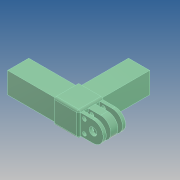
# Autodesk Inventor part: KB33-046-001-001 - Уголок
Saved by Autodesk Inventor 2020 (Build 240168000, 168)
## iProperties
Created: 2021-06-20
Part Number: KB33-046-001-001 - Уголок
Material: Пластик АБС
Document SubType Name: Modeling
Designer: Петров Иван
Mass: 150.443 g
Surface Area: 266.997 cm^2
Volume: 141.927 cm^3
Density: 1.06 g/cm^3
Appearance: Гладкий — темный цвет морской волны
Author: Петров Иван
Autodesk Inventor part; units mm, degrees
ref_plane "YZ Plane" through (0, 0, 0) normal (1, 0, 0) x (0, 1, 0)
ref_plane "XZ Plane" through (0, 0, 0) normal (0, 1, 0) x (-1, 0, 0)
ref_plane "XY Plane" through (0, 0, 0) normal (0, 0, 1) x (1, 0, 0)
sketch "Эскиз1" plane through (0, 0, 0) normal (0, 1, 0) x (-1, 0, 0)
  line L0 (-16, 16) -> (16, 16)
  line L1 (16, 16) -> (16, -16)
  line L2 (16, -16) -> (-16, -16)
  line L3 (-16, -16) -> (-16, 16)
  line L4 (-16, 16) -> (16, -16) construction
  line L5 (16, 16) -> (-16, -16) construction
  point P0 (0, 0)
  dimension "d0" = 32
  dimension "d1" = 32
  constraints: 12 end point, 2 midpoint, 2 parallel, 1 horizontal, 1 perpendicular
  measures "d0" distance of L1.end L2.end
  measures "d1" distance of L0.end L1.end
extrude "Выдавливание1" add sketch "Эскиз1" along normal blind 32
sketch "Эскиз2" plane through (16, 0, -16) normal (0, 0, -1) x (-1, 0, 0)
  line L0 (16, 0) -> (16, 16) construction
  line L1 (2, 2) -> (30, 2)
  line L2 (30, 2) -> (30, 30)
  line L3 (30, 30) -> (2, 30)
  line L4 (2, 30) -> (2, 2)
  line L5 (2, 2) -> (30, 30) construction
  line L6 (30, 2) -> (2, 30) construction
  dimension "d5" = 16
  dimension "d6" = 28
  dimension "d7" = 28
  constraints: 14 end point, 2 midpoint, 2 parallel, 1 horizontal, 1 perpendicular, 1 vertical
  measures "d5" distance of L0.start L0.end
  measures "d6" distance of L3.end L2.end
  measures "d7" distance of L2.end L1.end
extrude "Выдавливание2" add sketch "Эскиз2" along normal blind 64
pattern_circular "Круговой массив1" count 2 over 90 about axis through (0, -10, 0) along (0, 1, 0) of "Выдавливание2"
fillet "Сопряжение1" radius 2.5 5 edges at (16, 32, 0) (0, 32, 16) (0, 0, 16) (16, 0, 0) (16, 16, 16)
sketch "Эскиз5" plane through (16, 2.5, 13.5) normal (1, 0, 0) x (0, 0, -1)
  line L0 (0, 27) -> (29.5, 27) projected
  line L1 (0, 0) -> (0, 27) projected
  line L2 (29.5, 0) -> (0, 0) projected
  line L3 (29.5, 0) -> (29.5, 27) projected
  line L4 (0, 27) -> (29.5, 27) projected
  line L5 (29.5, 0) -> (0, 0) projected
  line L6 (0, 27) -> (4, 27)
  line L7 (4, 27) -> (4, 0)
  line L8 (4, 0) -> (0, 0)
  line L9 (0, 0) -> (0, 27)
  line L10 (29.5, 27) -> (25.5, 27)
  line L11 (25.5, 27) -> (25.5, 0)
  line L12 (25.5, 0) -> (29.5, 0)
  line L13 (29.5, 0) -> (29.5, 27)
  line L14 (10, 27) -> (19.5, 27)
  line L15 (19.5, 27) -> (19.5, 0)
  line L16 (19.5, 0) -> (10, 0)
  line L17 (10, 0) -> (10, 27)
  point P0 (13.5, -2.5)
  point P1 (10, 0)
  dimension "d14" = 4
  dimension "d15" = 4
  dimension "d16" = 6
  dimension "d17" = 6
  constraints: 24 end point, 6 parallel, 4 point on line, 3 horizontal, 3 perpendicular
  measures "d14" distance of L7.end L8.end
  measures "d15" distance of L12.end L11.end
  measures "d16" distance between parallel lines of L7 L17
  measures "d17" distance between parallel lines of L11 L15
extrude "Выдавливание3" add sketch "Эскиз5" along normal blind 30 contours L0 L7 L2 L1 | L0 L15 L2 L17 | L0 L3 L2 L11
fillet "Сопряжение2" radius 13.5 6 edges at (46, 29.5, 11.5) (46, 29.5, -1.25) (46, 29.5, -14) (46, 2.5, 11.5) (46, 2.5, -1.25) (46, 2.5, -14)
sketch "Эскиз6" plane through (16, 2.5, 13.5) normal (0, 0, 1) x (1, 0, 0)
  arc A0 (16.5, 0) -> (16.5, 27) centre (16.5, 13.5) ccw projected
  circle A1 centre (16.5, 13.5) radius 5
  point P0 (-16, -2.5)
  dimension "d21" = 10
  constraints: 1 centre point, 1 coincident
  measures "d21" diameter of A1
extrude "Выдавливание4" cut sketch "Эскиз6" against normal blind 59
sketch "Эскиз7" plane through (16, 2.5, 13.5) normal (0, 0, 1) x (1, 0, 0)
  circle A0 centre (5, 22) radius 2.5
  line L0 (0, 0) -> (0, 27) projected
  line L1 (0, 27) -> (16.5, 27) projected
  point P0 (-16, -2.5)
  dimension "d24" = 5
  dimension "d25" = 5
  dimension "d26" = 5
  constraints: 1 centre point
  measures "d24" diameter of A0
  measures "d25" distance from line of L0 A0.centre
  measures "d26" distance from line of L1 A0.centre
extrude "Выдавливание5" cut sketch "Эскиз7" against normal blind 59
ref_plane "РабПлоскость2" through (46, 16, 13.5) normal (0, 1, 0) x (1, 0, 0)
mirror "Зеркальное отражение1" about plane through (46, 16, 13.5) normal (0, 1, 0) of "Выдавливание5"
sketch "Эскиз8" plane through (16, 2.5, 3.5) normal (1, 0, 0) x (0, 0, -1)
  line L0 (-6, 27) -> (-6, 0) projected
  line L1 (0, 0) -> (0, 27) projected
  line L2 (-6, 22.5) -> (0, 22.5)
  line L3 (0, 22.5) -> (0, 4.5)
  line L4 (0, 4.5) -> (-6, 4.5)
  line L5 (-6, 4.5) -> (-6, 22.5)
  line L6 (-6, 27) -> (0, 27) projected
  line L7 (9.5, 27) -> (9.5, 0) projected
  line L8 (15.5, 0) -> (15.5, 27) projected
  line L9 (9.5, 22.5) -> (15.5, 22.5)
  line L10 (15.5, 22.5) -> (15.5, 4.5)
  line L11 (15.5, 4.5) -> (9.5, 4.5)
  line L12 (9.5, 4.5) -> (9.5, 22.5)
  point P0 (3.5, -2.5)
  point P1 (-6, 4.5)
  point P2 (0, 22.5)
  point P3 (12.5, 22.5)
  point P4 (-3, 22.5)
  point P5 (12.5, 4.5)
  point P6 (-3, 4.5)
  point P7 (9.5, 4.5)
  dimension "d29" = 18
  dimension "d30" = 4.5
  constraints: 16 end point, 4 midpoint, 4 parallel, 4 point on line, 2 horizontal, 2 horizontal alignment, 2 perpendicular
  measures "d29" distance between parallel lines of L4 L2
  measures "d30" distance between parallel lines of L6 L2
extrude "Выдавливание6" cut sketch "Эскиз8" against normal blind 8 contours L2 L1 L4 L0 | L9 L8 L11 L7
sketch "Эскиз9" plane through (16, 29.5, 3.5) normal (0, 0, 1) x (1, 0, 0)
  circle A0 centre (5, -22) radius 2.5 projected
  circle A1 centre (5, -5) radius 2.5 projected
  circle A2 centre (16.5, -13.5) radius 5 projected
  arc A3 (16.5, -27) -> (16.5, 0) centre (16.5, -13.5) ccw projected
  line L0 (0, 0) -> (16.5, 0) projected
  line L1 (0, -4.5) -> (0, 0) projected
  line L2 (0, -4.5) -> (-8, -4.5) projected
  line L3 (-8, -4.5) -> (-8, -22.5) projected
  line L4 (0, -22.5) -> (-8, -22.5) projected
  line L5 (0, -27) -> (0, -22.5) projected
  line L6 (0, -27) -> (16.5, -27) projected
  point P0 (-16, -29.5)
